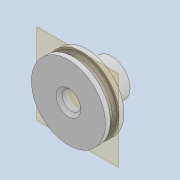
# Autodesk Inventor part: ned_s_1
Saved by Autodesk Inventor 2020 (Build 240168000, 168)
## iProperties
Created: 2021-10-09
Part Number: ned_s_1
Material: Generic
Document SubType Name: Modeling
Designer: Shuang Peng
Density: 1 g/cm^3
Appearance: Default
Author: Shuang Peng
Autodesk Inventor part; units mm, degrees
ref_plane "YZ Plane" through (0, 0, 0) normal (1, 0, 0) x (0, 1, 0)
ref_plane "XZ Plane" through (0, 0, 0) normal (0, 1, 0) x (-1, 0, 0)
ref_plane "XY Plane" through (0, 0, 0) normal (0, 0, 1) x (1, 0, 0)
sketch "Sketch1" plane through (0, 0, 0) normal (0, 0, 1) x (1, 0, 0)
  circle A0 centre (0, 0) radius 1.5
  circle A1 centre (0, 0) radius 3
  dimension "d0" = 3
  dimension "d1" = 6
  constraints: 2 centre point, 2 coincident
  measures "d0" diameter of A0
  measures "d1" diameter of A1
extrude "Extrusion1" add sketch "Sketch1" against normal blind 2
sketch "Sketch2" plane through (0, 0, -2) normal (0, 0, -1) x (-1, 0, 0)
  circle A0 centre (0, 0) radius 6
  circle A1 centre (0, 0) radius 1.5 projected
  dimension "d4" = 12
  constraints: 1 centre point, 1 coincident
  measures "d4" diameter of A0
extrude "Extrusion2" add sketch "Sketch2" along normal blind 3
sketch "Sketch3" plane through (0, 0, -5) normal (0, 0, -1) x (-1, 0, 0)
  circle A0 centre (0, 0) radius 1.5 projected
  circle A1 centre (0, 0) radius 1 projected
  circle A2 centre (0, 0) radius 1.5
  circle A3 centre (0, 0) radius 3
  point P0 (0, 0)
  dimension "d7" = 3
  dimension "d8" = 6
  constraints: 2 centre point, 2 coincident
  measures "d7" diameter of A2
  measures "d8" diameter of A3
extrude "Extrusion3" add sketch "Sketch3" along normal blind 2 contours A3
thicken "Thicken1" operation add thickness 2 both sides no extend neighbours yes toward (0, 0, -1) faces at (2.4709, -0.2393, 0)
ref_plane "Work Plane1" through (0, 0, -3.5) normal (0, 0, 1) x (1, 0, 0)
sketch "Sketch4" plane through (0, 0, -3.5) normal (0, 0, 1) x (1, 0, 0)
  circle A0 centre (0, 0) radius 6 projected
  circle A1 centre (0, 0) radius 5.3
  dimension "d14" = 0.7
  constraints: 1 centre point, 1 coincident
  measures "d14" radial gap between concentric circles of A0 A1
extrude "Extrusion4" cut sketch "Sketch4" against normal mid plane 1.4
fillet "Fillet1" radius 0.4 2 edges at (-5.3, 0, -2.8) (-5.3, 0, -4.2)
fillet "Fillet2" radius 1 1 edges at (3, 0, -5)
thicken "Thicken2" operation add thickness 2 both sides no extend neighbours yes toward (0, 0, -1) faces at (-2.4564, -0.359, -7)
chamfer "Chamfer2" distance 0.5 angle 45 2 edges at (1.5, 0, -9) (1.5, 0, -2)
body "Solid1"
